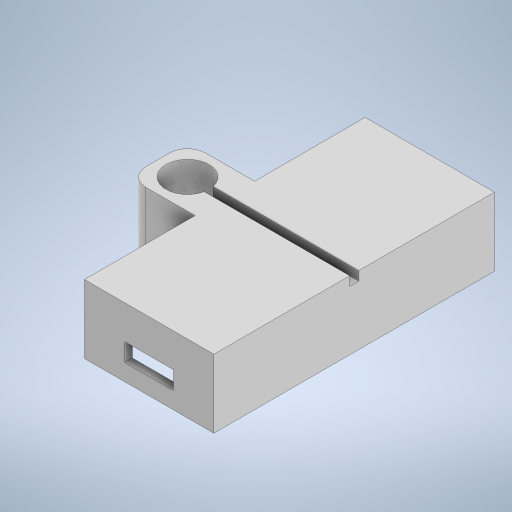
# Autodesk Inventor part: Arduino Mount
Saved by Autodesk Inventor 2024 (Build 280153000, 153)
## iProperties
Created: 2023-11-29
Part Number: Arduino Mount
Material: Generic
Document SubType Name: Modeling
Designer: close
Density: 1 g/cm^3
Appearance: Default
Author: close
Autodesk Inventor part; units mm, degrees
ref_plane "YZ Plane" through (0, 0, 0) normal (1, 0, 0) x (0, 1, 0)
ref_plane "XZ Plane" through (0, 0, 0) normal (0, 1, 0) x (-1, 0, 0)
ref_plane "XY Plane" through (0, 0, 0) normal (0, 0, 1) x (1, 0, 0)
sketch "Sketch1" plane through (0, 0, 0) normal (0, 1, 0) x (-1, 0, 0)
  line L0 (-7.5, 22.32) -> (-26.74, 22.32)
  line L1 (-26.74, 22.32) -> (-26.74, -22.32)
  line L2 (-26.74, -22.32) -> (-7.5, -22.32)
  line L3 (-7.5, -22.32) -> (-7.5, 22.32)
  line L4 (-7.5, 5) -> (2, 5)
  line L5 (5, 2) -> (5, -2)
  line L6 (2, -5) -> (-7.5, -5)
  line L7 (-7.5, -5) -> (-7.5, 5)
  line L8 (0, 0.75) -> (-7.5, 0.75)
  line L9 (-7.5, 0.75) -> (-7.5, -0.75)
  line L10 (-7.5, -0.75) -> (0, -0.75)
  line L11 (0, -0.75) -> (0, 0.75)
  circle A0 centre (0, 0) radius 3.625
  arc A1 (5, 2) -> (2, 5) centre (2, 2) ccw
  arc A2 (2, -5) -> (5, -2) centre (2, -2) ccw
  circle A3 centre (0, 0) radius 1.65
  line L12 (-9.5, 20.32) -> (-24.74, 20.32) construction
  line L13 (-24.74, 20.32) -> (-24.74, -20.32) construction
  line L14 (-24.74, -20.32) -> (-9.5, -20.32) construction
  line L15 (-9.5, -20.32) -> (-9.5, 20.32) construction
  circle A4 centre (-9.5, 20.32) radius 2
  circle A5 centre (-9.5, 20.32) radius 0.75
  circle A6 centre (-9.5, -20.32) radius 2
  circle A7 centre (-9.5, -20.32) radius 0.75
  circle A8 centre (-24.74, -20.32) radius 2
  circle A9 centre (-24.74, -20.32) radius 0.75
  circle A10 centre (-24.74, 20.32) radius 2
  circle A11 centre (-24.74, 20.32) radius 0.75
  line L16 (-27.99, -23.57) -> (-6.25, -23.57)
  line L17 (-6.25, -23.57) -> (-6.25, 23.57)
  line L18 (-6.25, 23.57) -> (-27.99, 23.57)
  line L19 (-27.99, 23.57) -> (-27.99, -23.57)
  line L20 (-7.5, 0.75) -> (-27.99, 0.75)
  line L21 (-27.99, 0.75) -> (-27.99, -0.75)
  line L22 (-27.99, -0.75) -> (-7.5, -0.75)
  line L23 (-7.5, -0.75) -> (-7.5, 0.75)
  point P0 (-6.25, -5)
  point P1 (-6.25, 5)
  point P2 (-3.5466, 0.75)
  point P3 (-3.5466, -0.75)
  point P4 (-27.99, 0)
  dimension "d2" = 10
  dimension "d3" = 12.5
  dimension "d4" = 7.25
  dimension "d5" = 1.5
  dimension "d6" = 0.75
  dimension "d7" = 0
  dimension "d8" = 5
  dimension "d10" = 5
  dimension "d11" = 3
  dimension "d12" = 3.3
  dimension "d13" = 40.64
  dimension "d14" = 15.24
  dimension "d15" = 1.5
  dimension "d16" = 4
  dimension "d17" = 1.25
  dimension "d18" = 1.25
  dimension "d19" = 1.25
  dimension "d20" = 1.25
  dimension "d21" = 20.32
  dimension "d25" = 0
  constraints: 48 end point, 12 centre point, 12 parallel, 11 coincident, 8 tangent, 7 equal radius, 6 horizontal, 6 perpendicular, 4 point on circle, 2 midpoint, 2 point on line, 1 collinear
  measures "d2" distance between parallel lines of L6 L4
  measures "d3" distance between parallel lines of L3 L5
  measures "d4" diameter of A0
  measures "d5" distance between parallel lines of L8 L10
  measures "d6" distance from line of point (0, 0) L10
  measures "d7" distance from line of point (0, 0) L11
  measures "d8" distance from line of point (0, 0) L5
  measures "d10" distance from line of point (0, 0) L4
  measures "d11" radius of A1
  measures "d12" diameter of A3
  measures "d13" distance of L14.end L12.start
  measures "d14" distance of L12.start L12.end
  measures "d15" diameter of A5
  measures "d16" diameter of A4
  measures "d17" distance between parallel lines of L3 L17
  measures "d18" distance between parallel lines of L18 L0
  measures "d19" distance between parallel lines of L16 L2
  measures "d20" distance between parallel lines of L1 L19
  measures "d21" vertical distance of point (0, 0) A4.centre
  measures "d25" distance from line of point (-27.99, 0) L19
extrude "Extrusion1" add sketch "Sketch1" along normal blind 1.5 contours L3 A4 L0 | L0 L1 L20 L19 L18 L17 L4 L3 | A4 L3 L20 L1 A10 L0 | A4 | A10 L1 L0 | A10 | L4 L17 L8 L3 | L4 A1 L5 A2 L6 L17 L10 A0 L8 | L10 L17 L6 L3 | L3 A6 L2 A8 L1 L22 | L1 L2 L3 L6 L17 L16 L19 L22 | A8 L2 L1 | A8 | A6 | L3 L2 A6 | A5 | A7 | A9 | A11
extrude "Extrusion2" add sketch "Sketch1" against normal blind 3.5 contours A4 | A10 | A8 | A6
extrude "Extrusion3" add sketch "Sketch1" against normal blind 1 contours L3 A4 L0 | L0 L1 L20 L19 L18 L17 L4 L3 | A4 L3 L20 L1 A10 L0 | A4 | A10 L1 L0 | A10 | L4 L17 L8 L3 | L8 L17 L10 L3 | L3 L22 L1 L20 | L1 L22 L19 L20 | L10 L17 L6 L3 | L3 A6 L2 A8 L1 L22 | L1 L2 L3 L6 L17 L16 L19 L22 | A8 L2 L1 | A8 | A6 | L3 L2 A6 | A5 | A7 | A9 | A11
extrude "Extrusion4" add sketch "Sketch1" against normal blind 9 contours L4 A1 L5 A2 L6 L17 L10 A0 L8 | L8 A0 L10 L17
extrude "Extrusion5" add sketch "Sketch1" against normal blind 10 contours L0 L1 L20 L19 L18 L17 L4 L3 | L4 L17 L8 L3 | L8 L17 L10 L3 | L1 L22 L19 L20 | L10 L17 L6 L3 | L1 L2 L3 L6 L17 L16 L19 L22
sketch "Sketch2" plane through (0, -9, 0) normal (0, -1, 0) x (1, 0, 0)
  circle A0 centre (0, 0) radius 3.625 projected
  circle A1 centre (0, 0) radius 1.65 projected
extrude "Extrusion6" add sketch "Sketch2" against normal blind 1
sketch "Sketch3" plane through (26.74, -10, 22.32) normal (0, 0, -1) x (-1, 0, 0)
  line L0 (17.99, 6.5) -> (16.49, 6.5) projected
  line L1 (2.75, 6.5) -> (1.25, 6.5) projected
  line L2 (13.695, 2.85) -> (5.545, 2.85)
  line L3 (5.545, 2.85) -> (5.545, 5.85)
  line L4 (5.545, 5.85) -> (13.695, 5.85)
  line L5 (13.695, 5.85) -> (13.695, 2.85)
  line L6 (-1.25, 0) -> (-1.25, 11.5) projected
  line L7 (20.49, 0) -> (20.49, 11.5) projected
  point P0 (26.74, 10)
  point P1 (13.695, 4.35)
  point P2 (2, 6.5)
  dimension "d36" = 8.15
  dimension "d37" = 3
  dimension "d38" = 21.74
  dimension "d39" = 6.795
  dimension "d42" = 0.65
  constraints: 8 end point, 2 midpoint, 2 parallel, 1 horizontal, 1 perpendicular
  measures "d36" distance between parallel lines of L3 L5
  measures "d37" distance between parallel lines of L4 L2
  measures "d38" distance between parallel lines of L6 L7
  measures "d39" distance from line of point (13.695, 4.35) L7
  measures "d42" distance from line of point (2, 6.5) L4
extrude "Extrusion7" cut sketch "Sketch3" against normal through all
equation "\"d2\" = 2 * d8"
equation "\"d6\" = 0.5 * d5"
equation "\"d10\" = d8"
equation "\"d18\" = d17"
equation "\"d19\" = d18"
equation "\"d20\" = d18"
equation "\"d21\" = 0.5 * d13"
equation "\"d39\" = -0.5 * d36 + 0.5 * d38"
body "Solid1"
